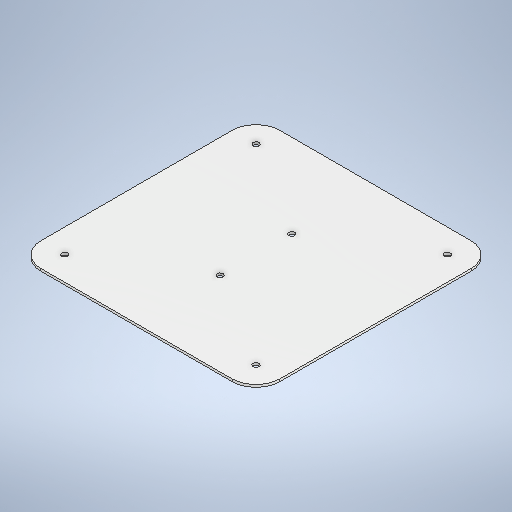
# Autodesk Inventor part: Basequadrada
Saved by Autodesk Inventor 2025 (Build 290162010, 162A)
## iProperties
Created: 2024-09-22
Part Number: Basequadrada
Material: PPS Plastic
Document SubType Name: Modeling
Designer: Bryan Ss
Density: 1.637 g/cm^3
Appearance: Smooth - White
Author: Bryan Ss
Autodesk Inventor part; units mm, degrees
ref_plane "YZ Plane" through (0, 0, 0) normal (1, 0, 0) x (0, 1, 0)
ref_plane "XZ Plane" through (0, 0, 0) normal (0, 1, 0) x (-1, 0, 0)
ref_plane "XY Plane" through (0, 0, 0) normal (0, 0, 1) x (1, 0, 0)
sketch "Sketch1" plane through (0, 0, 0) normal (0, 1, 0) x (-1, 0, 0)
  line L0 (0, 0) -> (200, 0)
  line L1 (200, 0) -> (200, -200)
  line L2 (200, -200) -> (0, -200)
  line L3 (0, -200) -> (0, 0)
  dimension "d0" = 200
  dimension "d1" = 200
  constraints: 8 end point, 2 parallel, 1 horizontal, 1 perpendicular
  measures "d0" distance of L1.end L2.end
  measures "d1" distance of L0.end L1.end
extrude "Extrusion1" add sketch "Sketch1" along normal blind 2
fillet "Fillet1" radius 20 4 edges at (-200, 1, 0) (0, 1, 0) (0, 1, -200) (-200, 1, -200)
sketch "Sketch4" plane through (0, 2, 0) normal (0, 1, 0) x (1, 0, 0)
  arc A0 (-20, 0) -> (0, 20) centre (-20, 20) ccw projected
  arc A1 (-200, 20) -> (-180, 0) centre (-180, 20) ccw projected
  arc A2 (0, 180) -> (-20, 200) centre (-20, 180) ccw projected
  arc A3 (-180, 200) -> (-200, 180) centre (-180, 180) ccw projected
  circle A4 centre (-20, 180) radius 2.5
  circle A5 centre (-180, 180) radius 2.5
  circle A6 centre (-180, 20) radius 2.5
  circle A7 centre (-20, 20) radius 2.5
  line L0 (-180, 0) -> (-20, 0) projected
  line L1 (0, 20) -> (0, 180) projected
  point P0 (0, 0)
  dimension "d19" = 5
  dimension "d20" = 5
  dimension "d21" = 5
  dimension "d22" = 5
  constraints: 4 centre point, 4 coincident
  measures "d19" diameter of A4
  measures "d20" diameter of A5
  measures "d21" diameter of A6
  measures "d22" diameter of A7
extrude "Extrusion4" cut sketch "Sketch4" against normal blind 2
sketch "Sketch6" plane through (0, 2, 0) normal (0, 1, 0) x (1, 0, 0)
  circle A0 centre (-100, 70) radius 2.5
  circle A1 centre (-100, 130) radius 2.5
  point P0 (0, 0)
  dimension "d34" = 5
  dimension "d35" = 5
  constraints: 2 centre point
  measures "d34" diameter of A0
  measures "d35" diameter of A1
extrude "Extrusion6" cut sketch "Sketch6" against normal blind 10
body "Solid1"
